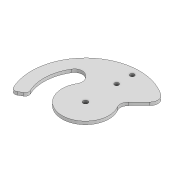
# Autodesk Inventor part: capstone hook constant radius
Saved by Autodesk Inventor 2020 (Build 240168000, 168)
## iProperties
Created: 2020-02-10
Part Number: capstone hook constant radius
Material: Generic
Document SubType Name: Modeling
Designer: ball
Density: 1 g/cm^3
Appearance: Default
Author: ball
Autodesk Inventor part; units mm, degrees
ref_plane "YZ Plane" through (0, 0, 0) normal (1, 0, 0) x (0, 1, 0)
ref_plane "XZ Plane" through (0, 0, 0) normal (0, 1, 0) x (-1, 0, 0)
ref_plane "XY Plane" through (0, 0, 0) normal (0, 0, 1) x (1, 0, 0)
sketch "Sketch1" plane through (0, 0, 0) normal (0, 1, 0) x (-1, 0, 0)
  arc A0 (28.8391, -17.7878) -> (30.6877, 14.3655) centre (0, 0) ccw
  arc A1 (-25.4519, -35.945) -> (39.7384, 18.992) centre (0, 0) ccw
  arc A2 (16.4102, -9.675) -> (-16.4102, -9.675) centre (0, 0) ccw
  line L0 (0, 0) -> (38.1429, 22.0218) construction
  line L1 (0, 0) -> (44.0436, 0) construction
  line L2 (31.9757, 18.4612) -> (35.2863, 20.3725)
  circle A3 centre (0, 0) radius 1.9304
  line L3 (0, 0) -> (31.1435, -31.1435) construction
  line L4 (0, 0) -> (44.0436, 0) construction
  line L5 (17.3902, -17.3902) -> (18.9443, -18.9443)
  line L6 (0, 0) -> (-26.2725, -26.2725) construction
  line L7 (0, 0) -> (37.1549, 0) construction
  line L8 (-17.3902, -17.3902) -> (-26.2725, -26.2725)
  arc A4 (39.7384, 18.992) -> (35.2863, 20.3725) centre (36.8738, 17.6229) ccw
  arc A5 (31.9757, 18.4612) -> (30.6877, 14.3655) centre (33.5632, 15.7115) ccw
  arc A6 (-26.2725, -26.2725) -> (-25.4519, -35.945) centre (-21.7823, -30.7626) ccw
  arc A7 (-17.3902, -17.3902) -> (-16.4102, -9.675) centre (-21.8803, -12.9001) ccw
  arc A8 (16.4102, -9.675) -> (17.3902, -17.3902) centre (21.8803, -12.9001) ccw
  arc A9 (18.9443, -18.9443) -> (28.8391, -17.7878) centre (23.4345, -14.4542) ccw
  circle A10 centre (0, -38.1) radius 1.7
  circle A11 centre (0, -25.4) radius 1.7
  point P0 (29.3441, 16.9418)
  point P1 (13.4704, -13.4704)
  point P2 (-13.4704, -13.4704)
  point P3 (23.9593, -23.9593)
  dimension "d0" = 67.7672
  dimension "d1" = 88.0872
  dimension "d2" = 38.1
  dimension "d3" = 30
  dimension "d4" = 3.8608
  dimension "d5" = 45
  dimension "d6" = 135
  dimension "d7" = 3.175
  dimension "d8" = 6.35
  dimension "d9" = 3.4
  dimension "d10" = 3.4
  dimension "d11" = 25.4
  dimension "d12" = 12.7
  constraints: 24 point on circle, 18 end point, 12 centre point, 12 tangent, 9 point on line, 4 coincident, 4 equal radius, 3 equal length, 3 horizontal, 1 collinear
  measures "d0" diameter of A0
  measures "d1" diameter of A1
  measures "d2" diameter of A2
  measures "d3" angle of L1 L0
  measures "d4" diameter of A3
  measures "d5" angle of L3 L4
  measures "d6" angle of L6 L7
  measures "d7" radius of A4
  measures "d8" radius of A6
  measures "d9" diameter of A10
  measures "d10" diameter of A11
  measures "d11" distance of A11.centre point (0, 0)
  measures "d12" distance of A10.centre A11.centre
extrude "Extrusion1" add sketch "Sketch1" along normal blind 2.54
body "Solid1"
